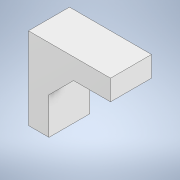
# Autodesk Inventor part: Soporte_cajas
Saved by Autodesk Inventor 2020 (Build 240168000, 168)
## iProperties
Created: 2020-11-04
Part Number: Soporte_cajas
Material: Plástico PC/ABS
Document SubType Name: Modeling
Designer: Cerberus 1S
Density: 0.357273 g/cm^3
Appearance: Suave - Blanco
Author: Cerberus 1S
Autodesk Inventor part; units mm, degrees
ref_plane "YZ Plane" through (0, 0, 0) normal (1, 0, 0) x (0, 1, 0)
ref_plane "XZ Plane" through (0, 0, 0) normal (0, 1, 0) x (-1, 0, 0)
ref_plane "XY Plane" through (0, 0, 0) normal (0, 0, 1) x (1, 0, 0)
sketch "Boceto1" plane through (0, 0, 0) normal (0, 0, 1) x (1, 0, 0)
  line L0 (0, 0) -> (0, 20)
  line L1 (0, 20) -> (20, 20)
  line L2 (20, 20) -> (20, 15)
  line L3 (20, 15) -> (5, 15)
  line L4 (5, 15) -> (5, 0)
  line L5 (5, 0) -> (0, 0)
  line L6 (0, 12.84) -> (-1.8, 12.84)
  line L7 (-1.8, 12.84) -> (-1.8, 15.5)
  line L8 (-1.8, 15.5) -> (-3.44, 15.5)
  line L9 (-3.44, 15.5) -> (-3.44, 4.5)
  line L10 (-3.44, 4.5) -> (-1.8, 4.5)
  line L11 (-1.8, 4.5) -> (-1.8, 7.16)
  line L12 (-1.8, 7.16) -> (0, 7.16)
  line L13 (0, 12.84) -> (0, 7.16)
  dimension "d0" = 20
  dimension "d1" = 20
  dimension "d2" = 5
  dimension "d3" = 5
  dimension "d7" = 11
  dimension "d8" = 1.8
  dimension "d9" = 1.64
  dimension "d10" = 5.68
  dimension "d11" = 2.66
  dimension "d12" = 2.66
  dimension "d13" = 7.16
  dimension "d14" = 7.16
  constraints: 28 end point, 11 perpendicular, 4 point on line, 1 collinear, 1 vertical
  measures "d0" distance of L0.start L0.end
  measures "d1" distance of L0.end L1.end
  measures "d2" distance between parallel lines of L0 L4
  measures "d3" distance between parallel lines of L1 L3
  measures "d7" distance of L8.end L9.end
  measures "d8" distance of L11.end L12.end
  measures "d9" distance between parallel lines of L9 L7
  measures "d10" distance between parallel lines of L12 L6
  measures "d11" distance between parallel lines of L8 L6
  measures "d12" distance between parallel lines of L10 L12
  measures "d13" distance between parallel lines of L5 L12
  measures "d14" distance between parallel lines of L1 L6
extrude "Extrusión1" add sketch "Boceto1" along normal blind 10 contours L0 L1 L2 L3 L4 L5
chamfer "Chaflán1" distance 6 angle 45 1 edges at (5, 15, 5)
equation "\"d11\" = d12"
equation "\"d13\" = d14"
